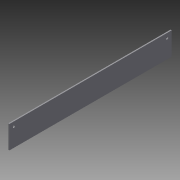
# Autodesk Inventor part: chain guard
Saved by Autodesk Inventor 2015 SP1 (Build 190203100, 203)
## iProperties
Created: 2015-01-17
Part Number: chain guard
Material: Generic
Document SubType Name: Modeling
Designer: Jarod
Density: 1 g/cm^3
Appearance: Default
Author: Jarod
Autodesk Inventor part; units mm, degrees
ref_plane "YZ Plane" through (0, 0, 0) normal (1, 0, 0) x (0, 1, 0)
ref_plane "XZ Plane" through (0, 0, 0) normal (0, 1, 0) x (-1, 0, 0)
ref_plane "XY Plane" through (0, 0, 0) normal (0, 0, 1) x (1, 0, 0)
sketch "Sketch1" plane through (0, 0, 0) normal (1, 0, 0) x (0, 1, 0)
  line L0 (0, 0) -> (63.5, 0)
  line L1 (63.5, 0) -> (63.5, -450.85)
  line L2 (63.5, -450.85) -> (0, -450.85)
  line L3 (0, -450.85) -> (0, 0)
  dimension "d0" = 63.5
  dimension "d1" = 450.85
  constraints: 8 end point, 2 parallel, 1 horizontal, 1 perpendicular
  measures "d0" distance of L1.end L2.end
  measures "d1" distance of L0.end L1.end
extrude "Extrusion1" add sketch "Sketch1" along normal blind 3.175
sketch "Sketch2" plane through (3.175, 0, 0) normal (1, 0, 0) x (0, 0, -1)
  line L0 (0, 63.5) -> (0, 0) projected
  line L1 (0, 0) -> (450.85, 0) projected
  line L2 (450.85, 0) -> (450.85, 63.5) projected
  line L3 (450.85, 63.5) -> (0, 63.5) projected
  point P0 (31.75, 50.8)
  point P1 (438.15, 50.8)
  dimension "d4" = 31.75
  dimension "d5" = 12.7
  dimension "d6" = 12.7
  dimension "d7" = 12.7
  measures "d4" distance from line of L0 point (31.75, 50.8)
  measures "d5" distance from line of L3 point (31.75, 50.8)
  measures "d6" distance from line of L2 point (438.15, 50.8)
  measures "d7" distance from line of L3 point (438.15, 50.8)
hole "Hole1" at (3.175, 50.8, -31.75) at (3.175, 50.8, -438.15) direction (-1, 0, 0) diameter 6.35 end through all
sketch "Sketch3" plane through (3.175, 0, 0) normal (1, 0, 0) x (0, 0, -1)
  circle A0 centre (31.75, 50.8) radius 3.175 projected
  circle A1 centre (438.15, 50.8) radius 3.175 projected
  line L0 (0, 63.5) -> (0, 0) projected
  line L1 (0, 0) -> (450.85, 0) projected
  line L2 (450.85, 0) -> (450.85, 63.5) projected
  line L3 (450.85, 63.5) -> (0, 63.5) projected
  line L4 (0, 0) -> (0, 38.1)
  line L5 (0, 0) -> (19.05, 0)
  line L6 (0, 0) -> (450.85, 0) projected
  line L7 (0, 38.1) -> (19.05, 0)
  dimension "d15" = 38.1
  dimension "d16" = 19.05
  constraints: 6 end point, 2 point on line
  measures "d15" distance of L0.end L4.end
  measures "d16" distance of L0.end L5.end
extrude "Extrusion2" cut sketch "Sketch3" against normal blind 3.175 contours L7 L1 L0
body "Solid1"
